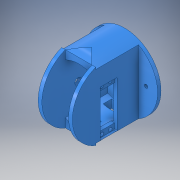
# Autodesk Inventor part: joint3_main
Saved by Autodesk Inventor 2019 (Build 230136000, 136)
## iProperties
Created: 2019-12-29
Part Number: joint3_main
Material: Пластик АБС
Document SubType Name: Modeling
Designer: Петров Иван
Density: 1.06 g/cm^3
Appearance: Голубой
Author: Петров Иван
Autodesk Inventor part; units mm, degrees
ref_plane "YZ Plane" through (0, 0, 0) normal (1, 0, 0) x (0, 1, 0)
ref_plane "XZ Plane" through (0, 0, 0) normal (0, 1, 0) x (-1, 0, 0)
ref_plane "XY Plane" through (0, 0, 0) normal (0, 0, 1) x (1, 0, 0)
sketch "Эскиз1" plane through (0, 0, 0) normal (0, 0, 1) x (1, 0, 0)
  circle A0 centre (29, 0) radius 2
  circle A1 centre (-29, 0) radius 2
  circle A2 centre (0, 8) radius 2
  circle A3 centre (8, 0) radius 2
  circle A4 centre (0, -8) radius 2
  circle A5 centre (-8, 0) radius 2
  circle A6 centre (0, 0) radius 42.5
  circle A7 centre (29, 0) radius 2
  circle A8 centre (-29, 0) radius 2
  circle A9 centre (0, 8) radius 2
  circle A10 centre (8, 0) radius 2
  circle A11 centre (0, -8) radius 2
  circle A12 centre (-8, 0) radius 2
  circle A13 centre (0, 0) radius 42.5
  constraints: 14 centre point
extrude "Выдавливание1" add sketch "Эскиз1" along normal blind 4
sketch "Эскиз16" plane through (0, 0, 4) normal (0, 0, 1) x (1, 0, 0)
  line L0 (-20, -37.5) -> (-20, 37.5)
  line L1 (20, 37.5) -> (20, -37.5)
  line L2 (20, -42.5) -> (-20, 42.5) construction
  line L3 (-20, -42.5) -> (20, 42.5) construction
  circle A0 centre (0, 0) radius 42.5 projected
  arc A1 (-20, -37.5) -> (20, -37.5) centre (0, 0) ccw
  arc A2 (20, 37.5) -> (-20, 37.5) centre (0, 0) ccw
  constraints: 8 end point, 8 point on circle, 2 centre point, 2 midpoint, 1 parallel
extrude "Выдавливание14" add sketch "Эскиз16" along normal blind 50 contours L0 A0 L1
sketch "Эскиз17" plane through (0, 0, 54) normal (0, 0, 1) x (1, 0, 0)
  line L0 (-15.66, -29.3625) -> (-15.66, 29.3625)
  line L1 (15.66, 29.3625) -> (15.66, -29.3625)
  line L2 (15.66, -33.2775) -> (-15.66, 33.2775) construction
  line L3 (-15.66, -33.2775) -> (15.66, 33.2775) construction
  arc A0 (-15.66, -29.3625) -> (15.66, -29.3625) centre (0, 0) ccw
  arc A1 (15.66, 29.3625) -> (-15.66, 29.3625) centre (0, 0) ccw
  arc A2 (-15.66, -29.3625) -> (15.66, -29.3625) centre (0, 0) ccw
  arc A3 (15.66, 29.3625) -> (-15.66, 29.3625) centre (0, 0) ccw
  constraints: 8 end point, 8 point on circle, 4 centre point, 2 midpoint, 1 parallel
extrude "Выдавливание15" cut sketch "Эскиз17" against normal up to surface (50 mm away)
sketch "Эскиз23" plane through (-20, -37.5, 4) normal (-1, 0, 0) x (0, 0, 1)
  line L0 (0, 39.5) -> (0, 35.5) projected
  line L1 (0, 37.5) -> (35, 37.5)
  circle A0 centre (35, 37.5) radius 3.9
  point P0 (-4, 37.5)
  dimension "d73" = 35
  dimension "d74" = 7.8
  constraints: 2 end point, 1 centre point, 1 coincident, 1 horizontal, 1 midpoint
  measures "d73" distance of L1.start L1.end
  measures "d74" diameter of A0
extrude "Выдавливание21" cut sketch "Эскиз23" against normal blind 54
sketch "Эскиз26" plane through (20, -37.5, 4) normal (1, 0, 0) x (0, 0, -1)
  circle A0 centre (-35, 37.5) radius 3.9 projected
  line L0 (-45, 47.5) -> (-25, 47.5)
  line L1 (-25, 47.5) -> (-25, 53.5)
  arc A1 (-25, 53.5) -> (-26, 54.5) centre (-26, 53.5) ccw
  line L2 (-26, 54.5) -> (-28.85, 54.5)
  line L3 (-28.85, 54.5) -> (-28.85, 53.434)
  arc A2 (-31.25, 53.434) -> (-28.85, 53.434) centre (-30.05, 51.65) ccw
  line L4 (-31.25, 53.434) -> (-31.25, 54.5)
  line L5 (-31.25, 54.5) -> (-38.75, 54.5)
  line L6 (-38.75, 54.5) -> (-38.75, 53.434)
  arc A3 (-41.15, 53.434) -> (-38.75, 53.434) centre (-39.95, 51.65) ccw
  line L7 (-41.15, 53.434) -> (-41.15, 54.5)
  line L8 (-41.15, 54.5) -> (-44, 54.5)
  arc A4 (-44, 54.5) -> (-45, 53.5) centre (-44, 53.5) ccw
  line L9 (-45, 53.5) -> (-45, 47.5)
  line L10 (-38.75, -0.2) -> (-38.75, 0.866)
  line L11 (-31.25, -0.2) -> (-38.75, -0.2)
  line L12 (-31.25, 0.866) -> (-31.25, -0.2)
  arc A5 (-28.85, 0.866) -> (-31.25, 0.866) centre (-30.05, 2.65) ccw
  line L13 (-28.85, -0.2) -> (-28.85, 0.866)
  line L14 (-26, -0.2) -> (-28.85, -0.2)
  arc A6 (-26, -0.2) -> (-25, 0.8) centre (-26, 0.8) ccw
  line L15 (-25, 6.8) -> (-25, 0.8)
  line L16 (-45, 6.8) -> (-25, 6.8)
  line L17 (-45, 0.8) -> (-45, 6.8)
  arc A7 (-45, 0.8) -> (-44, -0.2) centre (-44, 0.8) ccw
  line L18 (-41.15, -0.2) -> (-44, -0.2)
  line L19 (-41.15, 0.866) -> (-41.15, -0.2)
  arc A8 (-38.75, 0.866) -> (-41.15, 0.866) centre (-39.95, 2.65) ccw
  line L20 (-25, 47.5) -> (-25, 6.8)
  line L21 (-45, 6.8) -> (-45, 47.5)
  line L22 (-45, 47.5) -> (-25, 47.5)
  circle A9 centre (-35, 37.5) radius 1.25
  circle A10 centre (-35, 37.5) radius 3.4957
  circle A11 centre (-35, 37.5) radius 2.6787
  circle A12 centre (-35, 37.5) radius 5.4
  line L23 (-28.85, -0.2) -> (-31.25, -0.2)
  line L24 (-38.75, -0.2) -> (-41.15, -0.2)
  line L25 (-31.25, -0.2) -> (-34.5, -0.2)
  line L26 (-31.25, 54.5) -> (-38.75, 54.5)
  line L27 (-28.85, 54.5) -> (-31.25, 54.5)
  line L28 (-31.25, 54.5) -> (-38.75, 54.5)
  line L29 (-38.75, 54.5) -> (-41.15, 54.5)
  circle A13 centre (-30.05, 51.65) radius 2.15
  circle A14 centre (-39.95, 51.65) radius 2.15
  arc A15 (-38.75, 0.866) -> (-41.15, 0.866) centre (-39.95, 2.65) ccw
  circle A16 centre (-39.95, 2.65) radius 2.15
  circle A17 centre (-30.05, 2.65) radius 2.15
  circle A18 centre (-35, 37.5) radius 42.5
  line L30 (4, 80) -> (-50, 80) projected
  line L31 (-50, 0) -> (-50, -5) projected
  line L32 (-50, -2.2649) -> (-50, -5)
  line L33 (4, -5) -> (-50, -5) projected
  line L34 (-35, -5) -> (-50, -5)
  line L35 (4, -5) -> (-50, -5) projected
  line L36 (-50, 80) -> (-50, 75) projected
  line L37 (-50, 77.2649) -> (-50, 80)
  line L38 (-50, 80) -> (-35, 80)
  line L39 (4, 80) -> (-50, 80) projected
  point P0 (4, 37.5)
  point P1 (-45, 27.15)
  constraints: 68 end point, 22 point on circle, 17 centre point, 7 collinear, 5 coincident, 4 point on line, 2 concentric, 2 tangent, 3 other
extrude "Выдавливание23" cut sketch "Эскиз26" against normal blind 10 contours A0 | L0 L20 L16 L21 | A9 | A10 | A11 | A12
sketch "Эскиз27" plane through (20, -37.5, 4) normal (1, 0, 0) x (0, 0, -1)
  circle A0 centre (-35, 37.5) radius 3.9
  line L0 (-45, 47.5) -> (-25, 47.5)
  line L1 (-25, 47.5) -> (-25, 53.5)
  arc A1 (-25, 53.5) -> (-26, 54.5) centre (-26, 53.5) ccw
  line L2 (-26, 54.5) -> (-28.85, 54.5)
  line L3 (-28.85, 54.5) -> (-28.85, 53.434)
  arc A2 (-31.25, 53.434) -> (-28.85, 53.434) centre (-30.05, 51.65) ccw
  line L4 (-31.25, 53.434) -> (-31.25, 54.5)
  line L5 (-31.25, 54.5) -> (-38.75, 54.5)
  line L6 (-38.75, 54.5) -> (-38.75, 53.434)
  arc A3 (-41.15, 53.434) -> (-38.75, 53.434) centre (-39.95, 51.65) ccw
  line L7 (-41.15, 53.434) -> (-41.15, 54.5)
  line L8 (-41.15, 54.5) -> (-44, 54.5)
  arc A4 (-44, 54.5) -> (-45, 53.5) centre (-44, 53.5) ccw
  line L9 (-45, 53.5) -> (-45, 47.5)
  line L10 (-38.75, -0.2) -> (-38.75, 0.866)
  line L11 (-31.25, -0.2) -> (-38.75, -0.2)
  line L12 (-31.25, 0.866) -> (-31.25, -0.2)
  arc A5 (-28.85, 0.866) -> (-31.25, 0.866) centre (-30.05, 2.65) ccw
  line L13 (-28.85, -0.2) -> (-28.85, 0.866)
  line L14 (-26, -0.2) -> (-28.85, -0.2)
  arc A6 (-26, -0.2) -> (-25, 0.8) centre (-26, 0.8) ccw
  line L15 (-25, 6.8) -> (-25, 0.8)
  line L16 (-45, 6.8) -> (-25, 6.8)
  line L17 (-45, 0.8) -> (-45, 6.8)
  arc A7 (-45, 0.8) -> (-44, -0.2) centre (-44, 0.8) ccw
  line L18 (-41.15, -0.2) -> (-44, -0.2)
  line L19 (-41.15, 0.866) -> (-41.15, -0.2)
  arc A8 (-38.75, 0.866) -> (-41.15, 0.866) centre (-39.95, 2.65) ccw
  line L20 (-25, 47.5) -> (-25, 6.8)
  line L21 (-45, 6.8) -> (-45, 47.5)
  line L22 (-45, 47.5) -> (-25, 47.5)
  circle A9 centre (-35, 37.5) radius 1.25
  circle A10 centre (-35, 37.5) radius 3.4957
  circle A11 centre (-35, 37.5) radius 2.6787
  circle A12 centre (-35, 37.5) radius 5.4
  line L23 (-28.85, -0.2) -> (-31.25, -0.2)
  line L24 (-38.75, -0.2) -> (-41.15, -0.2)
  line L25 (-31.25, -0.2) -> (-34.5, -0.2)
  line L26 (-31.25, 54.5) -> (-38.75, 54.5)
  line L27 (-28.85, 54.5) -> (-31.25, 54.5)
  line L28 (-31.25, 54.5) -> (-38.75, 54.5)
  line L29 (-38.75, 54.5) -> (-41.15, 54.5)
  circle A13 centre (-30.05, 51.65) radius 2.15
  circle A14 centre (-39.95, 51.65) radius 2.15
  arc A15 (-38.75, 0.866) -> (-41.15, 0.866) centre (-39.95, 2.65) ccw
  circle A16 centre (-39.95, 2.65) radius 2.15
  circle A17 centre (-30.05, 2.65) radius 2.15
  point P0 (4, 37.5)
  point P1 (4, 37.5)
  point P2 (-45, 27.15)
  constraints: 60 end point, 18 point on circle, 17 centre point, 4 coincident, 4 collinear, 2 concentric, 3 other
extrude "Выдавливание24" cut sketch "Эскиз27" against normal blind 3 contours L9 A4 L8 L7 A3 L6 L5 L4 A2 L3 L2 A1 L1 L0 | L16 L15 A6 L14 L13 A5 L12 L11 L10 A8 L19 L18 A7 L17 | L29 L6 A14 L7 | L3 A13 L4 L27 | A14 A3 | L19 A16 L10 L24 | A2 A13 | L23 L12 A17 L13 | A8 A16 | A17 A5
sketch "Эскиз28" plane through (17, -37.5, 4) normal (1, 0, 0) x (0, 0, -1)
  circle A0 centre (-35, 37.5) radius 3.9
  line L0 (-45, 47.5) -> (-25, 47.5)
  line L1 (-25, 47.5) -> (-25, 53.5)
  arc A1 (-25, 53.5) -> (-26, 54.5) centre (-26, 53.5) ccw
  line L2 (-26, 54.5) -> (-28.85, 54.5)
  line L3 (-28.85, 54.5) -> (-28.85, 53.434)
  arc A2 (-31.25, 53.434) -> (-28.85, 53.434) centre (-30.05, 51.65) ccw
  line L4 (-31.25, 53.434) -> (-31.25, 54.5)
  line L5 (-31.25, 54.5) -> (-38.75, 54.5)
  line L6 (-38.75, 54.5) -> (-38.75, 53.434)
  arc A3 (-41.15, 53.434) -> (-38.75, 53.434) centre (-39.95, 51.65) ccw
  line L7 (-41.15, 53.434) -> (-41.15, 54.5)
  line L8 (-41.15, 54.5) -> (-44, 54.5)
  arc A4 (-44, 54.5) -> (-45, 53.5) centre (-44, 53.5) ccw
  line L9 (-45, 53.5) -> (-45, 47.5)
  line L10 (-38.75, -0.2) -> (-38.75, 0.866)
  line L11 (-31.25, -0.2) -> (-38.75, -0.2)
  line L12 (-31.25, 0.866) -> (-31.25, -0.2)
  arc A5 (-28.85, 0.866) -> (-31.25, 0.866) centre (-30.05, 2.65) ccw
  line L13 (-28.85, -0.2) -> (-28.85, 0.866)
  line L14 (-26, -0.2) -> (-28.85, -0.2)
  arc A6 (-26, -0.2) -> (-25, 0.8) centre (-26, 0.8) ccw
  line L15 (-25, 6.8) -> (-25, 0.8)
  line L16 (-45, 6.8) -> (-25, 6.8)
  line L17 (-45, 0.8) -> (-45, 6.8)
  arc A7 (-45, 0.8) -> (-44, -0.2) centre (-44, 0.8) ccw
  line L18 (-41.15, -0.2) -> (-44, -0.2)
  line L19 (-41.15, 0.866) -> (-41.15, -0.2)
  arc A8 (-38.75, 0.866) -> (-41.15, 0.866) centre (-39.95, 2.65) ccw
  line L20 (-25, 47.5) -> (-25, 6.8)
  line L21 (-45, 6.8) -> (-45, 47.5)
  line L22 (-45, 47.5) -> (-25, 47.5)
  circle A9 centre (-35, 37.5) radius 1.25
  circle A10 centre (-35, 37.5) radius 3.4957
  circle A11 centre (-35, 37.5) radius 2.6787
  circle A12 centre (-35, 37.5) radius 5.4
  line L23 (-28.85, -0.2) -> (-31.25, -0.2)
  line L24 (-38.75, -0.2) -> (-41.15, -0.2)
  line L25 (-31.25, -0.2) -> (-34.5, -0.2)
  line L26 (-31.25, 54.5) -> (-38.75, 54.5)
  line L27 (-28.85, 54.5) -> (-31.25, 54.5)
  line L28 (-31.25, 54.5) -> (-38.75, 54.5)
  line L29 (-38.75, 54.5) -> (-41.15, 54.5)
  circle A13 centre (-30.05, 51.65) radius 2.15
  circle A14 centre (-39.95, 51.65) radius 2.15
  arc A15 (-38.75, 0.866) -> (-41.15, 0.866) centre (-39.95, 2.65) ccw
  circle A16 centre (-39.95, 2.65) radius 2.15
  circle A17 centre (-30.05, 2.65) radius 2.15
  point P0 (4, 37.5)
  point P1 (4, 37.5)
  point P2 (-45, 27.15)
  constraints: 60 end point, 18 point on circle, 17 centre point, 4 coincident, 4 collinear, 2 concentric, 3 other
extrude "Выдавливание25" cut sketch "Эскиз28" against normal blind 15 contours A14 A3 | A2 A13 | A8 A16 | A17 A5
sketch "Эскиз29" plane through (20, -37.5, 4) normal (1, 0, 0) x (0, 0, -1)
  circle A0 centre (-35, 37.5) radius 3.9 projected
  circle A1 centre (-35, 37.5) radius 42.5
  line L0 (4, 80) -> (-50, 80) projected
  line L1 (-50, -2.2649) -> (-50, -5)
  line L2 (-50, -5) -> (-35, -5)
  line L3 (4, -5) -> (-50, -5) projected
  line L4 (-50, 80) -> (-50, 75) projected
  line L5 (-50, 77.2649) -> (-50, 80)
  line L6 (-50, 80) -> (-35, 80)
  point P0 (4, 37.5)
  constraints: 8 end point, 4 point on circle, 3 point on line, 1 centre point, 1 coincident, 1 collinear, 1 tangent, 1 vertical
extrude "Выдавливание26" cut sketch "Эскиз29" against normal blind 46.75 contours A1 L4 L0 | L2 L1 A1
sketch "Эскиз30" plane through (20, -37.5, 4) normal (1, 0, 0) x (0, 0, -1)
  circle A0 centre (-35, 37.5) radius 3.9 projected
  circle A1 centre (-35, 37.5) radius 42.5
  line L0 (-50, 0) -> (-50, -2.2649) projected
  line L1 (-50, -2.2649) -> (-50, 77.2649)
  line L2 (-50, 8.1375) -> (-50, 66.8625) projected
  point P0 (4, 37.5)
  constraints: 2 end point, 1 centre point, 1 coincident, 1 collinear, 1 point on circle
extrude "Выдавливание27" add sketch "Эскиз30" against normal up to surface (4.34 mm away) contours L1 L0 A1 picked at (-59.1667, 37.5)
sketch "Эскиз31" plane through (-20, -37.5, 4) normal (-1, 0, 0) x (0, 0, 1)
  circle A0 centre (35, 37.5) radius 3.9
  circle A1 centre (35, 37.5) radius 42.5
  line L0 (50, 75) -> (50, 77.2649)
  line L1 (50, 77.2649) -> (50, -2.2649)
  line L2 (50, 66.8625) -> (50, 8.1375)
  circle A2 centre (35, 37.5) radius 3.9 projected
  point P0 (-4, 37.5)
  point P1 (-4, 37.5)
  constraints: 6 end point, 2 centre point, 1 coincident, 1 collinear, 1 point on circle
extrude "Выдавливание28" add sketch "Эскиз31" against normal up to surface (4.34 mm away) contours A1 L1 L0 picked at (59.1667, 37.5)
sketch "Эскиз32" plane through (-20, -37.5, 4) normal (-1, 0, 0) x (0, 0, 1)
  circle A0 centre (35, 37.5) radius 3.9 projected
  line L0 (0, 0) -> (0, 75) projected
  line L1 (0, 0) -> (50, 0) projected
  line L2 (50, 0) -> (50, -2.2649) projected
  arc A1 (50, -2.2649) -> (50, 77.2649) centre (35, 37.5) ccw projected
  line L3 (50, 77.2649) -> (50, 75) projected
  line L4 (0, 75) -> (50, 75) projected
  point P0 (-4, 37.5)
ref_plane "РабПлоскость2" through (0, -42.5, 39) normal (0, -1, 0) x (1, 0, 0)
sketch "Эскиз33" plane through (0, -42.5, 39) normal (0, -1, 0) x (1, 0, 0)
  line L0 (-10, -33.6111) -> (10, -33.6111)
  line L1 (10, -33.6111) -> (10, -23.6111)
  line L2 (10, -23.6111) -> (-10, -23.6111)
  line L3 (-10, -23.6111) -> (-10, -33.6111)
  line L4 (-10, -33.6111) -> (10, -23.6111) construction
  line L5 (10, -33.6111) -> (-10, -23.6111) construction
  point P0 (0, -39)
  point P1 (0, -28.6111)
  dimension "d92" = 20
  dimension "d93" = 10
  constraints: 12 end point, 2 midpoint, 2 parallel, 1 horizontal, 1 perpendicular
  measures "d92" distance of L2.end L1.end
  measures "d93" distance of L1.end L0.end
extrude "Выдавливание29" cut sketch "Эскиз33" against normal blind 18.75
